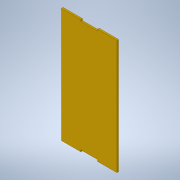
# Autodesk Inventor part: Part2
Saved by Autodesk Inventor 2020 (Build 240168000, 168)
## iProperties
Created: 2020-03-09
Part Number: Part2
Material: Generic
Document SubType Name: Modeling
Designer: tor16003
Density: 1 g/cm^3
Appearance: Gold
Author: tor16003
Autodesk Inventor part; units mm, degrees
ref_plane "YZ Plane" through (0, 0, 0) normal (1, 0, 0) x (0, 1, 0)
ref_plane "XZ Plane" through (0, 0, 0) normal (0, 1, 0) x (-1, 0, 0)
ref_plane "XY Plane" through (0, 0, 0) normal (0, 0, 1) x (1, 0, 0)
sketch "Sketch1" plane through (0, 0, 0) normal (0, 0, 1) x (1, 0, 0)
  line L0 (0, 0) -> (0, 206)
  line L1 (0, 206) -> (35, 206)
  line L2 (35, 206) -> (35, 203)
  line L3 (35, 203) -> (65, 203)
  line L4 (65, 203) -> (65, 206)
  line L5 (65, 206) -> (100, 206)
  line L6 (100, 206) -> (100, 0)
  line L7 (100, 0) -> (65, 0)
  line L8 (65, 0) -> (65, 3)
  line L9 (65, 3) -> (35, 3)
  line L10 (35, 3) -> (35, 0)
  line L11 (35, 0) -> (0, 0)
  dimension "d27" = 3
  dimension "d28" = 30
  dimension "d41" = 100
  dimension "d42" = 35
  dimension "d43" = 3
  dimension "d44" = 200
  constraints: 25 end point, 8 perpendicular, 3 point on line, 2 collinear, 2 vertical, 1 parallel
  measures "d27" distance of L7.end L8.end
  measures "d28" distance of L8.end L9.end
  measures "d41" distance between parallel lines of L0 L6
  measures "d42" distance between parallel lines of L0 L10
  measures "d43" distance between parallel lines of L3 L1
  measures "d44" distance between parallel lines of L9 L3
extrude "Extrusion1" add sketch "Sketch1" along normal blind 3
body "Solid1"
